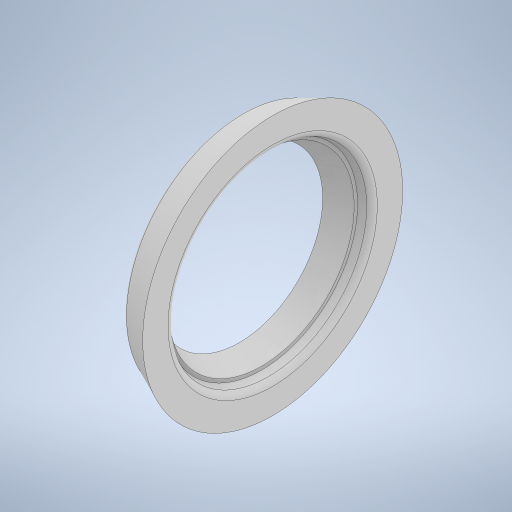
# Autodesk Inventor part: RangeHoodLightRing
Saved by Autodesk Inventor 2023 (Build 270158000, 158)
## iProperties
Created: 2023-05-30
Part Number: RangeHoodLightRing
Material: Generic
Document SubType Name: Modeling
Designer: lidang
Density: 1 g/cm^3
Appearance: Default
Author: lidang
## iProperties of the stored document RangeHoodLightRing_3DPrint.ipt
Created: 2023-05-30
Part Number: RangeHoodLightRing_3DPrint
Material: Generic
Document SubType Name: Modeling
Designer: lidang
Density: 1 g/cm^3
Appearance: Default
Author: lidang
Autodesk Inventor part; units mm, degrees
ref_plane "YZ Plane" through (0, 0, 0) normal (1, 0, 0) x (0, 1, 0)
ref_plane "XZ Plane" through (0, 0, 0) normal (0, 1, 0) x (-1, 0, 0)
ref_plane "XY Plane" through (0, 0, 0) normal (0, 0, 1) x (1, 0, 0)
sketch "Sketch1" plane through (0, 0, 0) normal (0, 1, 0) x (-1, 0, 0)
  line L0 (0, 0) -> (0, 29)
  line L1 (0, 29) -> (0, 30)
  line L2 (0, 39) -> (10, 34.5)
  line L3 (10, 0) -> (0, 0)
  line L4 (10, 0) -> (10, 25)
  line L5 (10, 25) -> (10, 34.5)
  line L6 (10, 25) -> (3.3, 27.7732)
  line L7 (3.3, 27.7732) -> (3.3, 28.7732)
  line L8 (3.3, 28.7732) -> (0, 30)
  line L9 (3.3, 27.7732) -> (0, 29)
  line L10 (0, 30) -> (0, 39)
  dimension "d0" = 29
  dimension "d1" = 10
  dimension "d2" = 25
  dimension "d3" = 9.5
  dimension "d4" = 3.3
  dimension "d5" = 30
  dimension "d7" = 10
  constraints: 22 end point, 5 vertical, 1 collinear, 1 parallel
  measures "d0" distance of L0.start L0.end
  measures "d1" distance of L0.end L2.start
  measures "d2" distance of L3.start L4.end
  measures "d3" distance of L4.end L2.end
  measures "d4" horizontal distance of L0.start L6.end
  measures "d5" distance of L0.start L1.end
  measures "d7" distance of L3.start L0.start
revolve "Revolution1" add sketch "Sketch1" angle 360 about axis through (-10, 0, 0) along (1, 0, 0) contours L10 L2 L5 L6 L7 L8
fillet "Fillet1" radius 2 1 edges at (-10, 0, -34.5)
fillet "Fillet2" radius 2 1 edges at (0, 0, -30)
body "Solid1"
